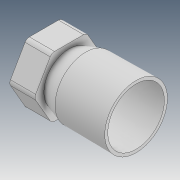
# Autodesk Inventor part: PneumaticAdaptorFemale
Saved by Autodesk Inventor 2020 (Build 240168000, 168)
## iProperties
Created: 2020-04-22
Part Number: PneumaticAdaptorFemale
Material: Generic
Document SubType Name: Modeling
Designer: Theo Cominotto
Density: 1 g/cm^3
Appearance: Default
Author: Theo Cominotto
Autodesk Inventor part; units mm, degrees
ref_plane "YZ Plane" through (0, 0, 0) normal (1, 0, 0) x (0, 1, 0)
ref_plane "XZ Plane" through (0, 0, 0) normal (0, 1, 0) x (-1, 0, 0)
ref_plane "XY Plane" through (0, 0, 0) normal (0, 0, 1) x (1, 0, 0)
sketch "Sketch1" plane through (0, 0, 0) normal (0, 0, 1) x (1, 0, 0)
  line L0 (0, 0) -> (6.6144, 0) construction
  line L1 (0, 0) -> (0, 4.75) construction
  line L2 (0, 4.75) -> (8, 4.3864)
  line L3 (6.6144, 0) -> (16.6144, 0) construction
  line L4 (16.6144, 0) -> (16.6144, 12.2) construction
  line L5 (16.6144, 0) -> (36.6144, 0) construction
  line L6 (36.6144, 0) -> (36.6144, 12.45) construction
  line L7 (36.6144, 12.45) -> (16.6144, 12.2)
  line L8 (0, 4.75) -> (0, 6.75)
  line L9 (0, 4.75) -> (2, 4.75) construction
  line L10 (0, 6.75) -> (16.6144, 12.2)
  line L11 (8, 4.3864) -> (16.6144, 11)
  line L12 (16.6144, 11) -> (36.6144, 11.2499)
  line L13 (36.6144, 11.2499) -> (36.6144, 12.45)
  line L14 (0, 0) -> (3.3, 0) construction
  line L15 (3.3, 0) -> (3.3, 4.6) construction
  dimension "d2" = 4.75
  dimension "d3" = 12.2
  dimension "d4" = 20
  dimension "d5" = 12.45
  dimension "d6" = 2
  dimension "d7" = 90
  dimension "d8" = 1.2
  dimension "d9" = 1.2
  dimension "d10" = 10
  dimension "d24" = 177.397
  dimension "d25" = 8
  dimension "d26" = 3.3
  dimension "d27" = 4.6
  dimension "d28" = 6.6144
  constraints: 32 end point, 4 horizontal, 4 point on line, 3 perpendicular, 2 vertical, 1 collinear
  measures "d2" distance of L0.start L1.end
  measures "d3" distance of L3.end L4.end
  measures "d4" distance of L3.end L5.end
  measures "d5" distance of L5.end L6.end
  measures "d6" distance of L1.end L8.end
  measures "d7" angle of L9 L8
  measures "d8" distance from line of L7 L12.end
  measures "d9" distance of L4.end L11.end
  measures "d10" distance of L0.end L3.end
  measures "d24" angle of L9 L2
  measures "d25" distance from line of L1 L2.end
  measures "d26" distance of L0.start L14.end
  measures "d27" distance of L14.end L15.end
  measures "d28" distance of L0.start L0.end
revolve "Revolution1" add sketch "Sketch1" angle 360 about axis through (6.6144, 0, 0) along (1, 0, 0)
sketch "Sketch2" plane through (0, 0, 0) normal (-1, 0, 0) x (0, 0, 1)
  circle A0 centre (0, 0) radius 6.75 projected
  line L0 (0, -6.75) -> (0, -12.2) construction
  circle A1 centre (0, 0) radius 12.2 projected
  line L1 (1.633, -6.5495) -> (2.9514, -11.8376)
  line L2 (-1.633, -6.5495) -> (-2.9514, -11.8376)
  point P0 (-1.633, -6.5495)
  point P1 (-2.9514, -11.8376)
  dimension "d12" = 14
  constraints: 6 end point, 4 point on circle, 2 symmetric about line, 1 point on line, 1 vertical
  measures "d12" angle of L0 L1
extrude "Extrusion1" [suppressed]
chamfer "Chamfer1" [suppressed]
pattern_circular "Circular Pattern1" [suppressed]
chamfer "Chamfer2" distance 0.7 angle 45 1 edges at (0, -4.75, 0)
sketch "Sketch3" plane through (0, 0, 0) normal (-1, 0, 0) x (0, 0, 1)
  line L0 (-6.9282, -12) -> (-13.8564, 0)
  line L1 (-13.8564, 0) -> (-6.9282, 12)
  line L2 (-6.9282, 12) -> (6.9282, 12)
  line L3 (6.9282, 12) -> (13.8564, 0)
  line L4 (13.8564, 0) -> (6.9282, -12)
  line L5 (6.9282, -12) -> (-6.9282, -12)
  circle A0 centre (0, 0) radius 6.75 projected
  point P0 (0, -12)
  dimension "d32" = 24
  constraints: 12 end point, 1 coincident, 1 midpoint, 13 other
  measures "d32" distance between parallel lines of L2 L5
extrude "Extrusion2" add sketch "Sketch3" against normal blind 10
fillet "Fillet1" radius 2 6 edges at (5, 12, 6.9282) (5, 12, -6.9282) (5, 0, -13.8564) (5, -12, -6.9282) (5, -12, 6.9282) (5, 0, 13.8564)
equation "\"Tol\" = 0"
body "Solid1"
